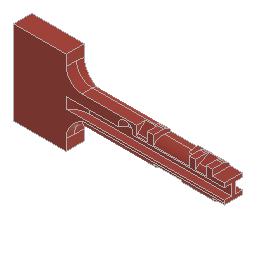
exec (Autodesk Fusion 360 design; units mm, degrees)
Autodesk Fusion 360 part; units mm, degrees
sketch "profile" plane through (0, 0, 0) normal (1, 0, 0) x (0, 1, 0)
  line L0 (0, 0) -> (1.725, 0) construction
  line L1 (1.725, 0) -> (1.725, 2.975) construction
  line L2 (0, 0) -> (1.5, 1.5) construction
  line L3 (0, 0) -> (1.725, 0) construction
  line L4 (1.725, 2.975) -> (1.725, 5.95) construction
  line L5 (1.725, 5.95) -> (3.45, 5.95) construction
  line L6 (3.45, 5.95) -> (1.95, 4.45) construction
  line L7 (1.725, 2.975) -> (1.375, 2.975) construction
  line L8 (1.375, 2.975) -> (1.375, 4)
  line L9 (1.725, 2.975) -> (2.075, 2.975) construction
  line L10 (1.375, 2.975) -> (1.375, 1.95)
  line L11 (2.075, 2.975) -> (2.075, 4)
  line L12 (2.075, 2.975) -> (2.075, 1.95)
  line L13 (1.375, 4) -> (0, 4)
  line L14 (1.375, 1.95) -> (0, 1.95)
  line L15 (2.075, 4) -> (3.45, 4)
  line L16 (2.075, 1.95) -> (3.45, 1.95)
  line L17 (3.45, 1.95) -> (3.45, 0)
  line L18 (0, 4) -> (0, 5.95)
  arc A0 (0, 1.5) -> (1.5, 0) centre (1.5, 1.5) ccw
  line L19 (0, 1.95) -> (0, 1.5)
  line L20 (1.5, 0) -> (3.45, 0)
  arc A1 (3.45, 4.45) -> (1.95, 5.95) centre (1.95, 4.45) ccw
  line L21 (1.95, 5.95) -> (0, 5.95)
  line L22 (3.45, 4.45) -> (3.45, 4)
  dimension "d1" = 1.725
  dimension "d2" = 2.975
  dimension "d3" = 45
  dimension "d4" = 2.1213
  dimension "d5" = 2.975
  dimension "d6" = 1.725
  dimension "d7" = 0.35
  dimension "d8" = 1.025
  dimension "d9" = 1.375
  constraint coincident L0.start L2.start
  constraint horizontal L0
  constraint perpendicular L0 L1
  constraint horizontal L3
  constraint parallel L1 L4
  constraint perpendicular L4 L5
  constraint equal L2 L6
  constraint parallel L2 L6
  constraint perpendicular L1 L7
  constraint perpendicular L7 L8
  constraint perpendicular L4 L9
  constraint equal L7 L9
  constraint perpendicular L7 L10
  constraint perpendicular L9 L11
  constraint perpendicular L9 L12
  constraint equal L8 L10
  constraint equal L10 L12
  constraint equal L11 L12
  constraint perpendicular L8 L13
  constraint perpendicular L10 L14
  constraint perpendicular L11 L15
  constraint perpendicular L12 L16
  constraint perpendicular L3 L17
  constraint perpendicular L5 L18
  constraint coincident L3 A0.end
  constraint coincident L2.end A0.centre
  constraint tangent A0 L19
  constraint tangent A0 L20
  constraint coincident L5 A1.end
  constraint coincident L6.end A1.centre
  constraint tangent A1 L21
  constraint tangent A1 L22
  constraint equal L13 L15
  constraint equal L15 L16
  constraint equal L14 L16
  constraint perpendicular L15 L22
  constraint parallel L20 L21
  measures "d1" distance of L0.start L0.end
  measures "d2" distance of L0.end L1.end
  measures "d3" angle of L2 L3
  measures "d4" distance of L0.start L2.end
  measures "d5" distance of L1.end L4.end
  measures "d6" distance of L4.end L5.end
  measures "d7" distance of L1.end L7.end
  measures "d8" distance of L7.end L8.end
  measures "d9" distance of L8.end L13.end
extrude "Extrude1" add sketch "profile" against normal blind 30
ref_plane "WorkPlane2" through (-30, 0, 0) normal (1, 0, 0) x (0, 1, 0)
sketch "bow" plane through (-30, 0, 0) normal (1, 0, 0) x (0, 1, 0)
  line L0 (0, 0) -> (0, -5.025)
  line L1 (0, 0) -> (0, 10.975)
  line L2 (0, 10.975) -> (3.45, 10.975)
  line L3 (3.45, 10.975) -> (3.45, -5.025)
  line L4 (3.45, -5.025) -> (0, -5.025)
  dimension "d91" = 5.025
  dimension "d92" = 10.975
  dimension "d93" = 3.45
  constraint coincident L0.start L1.start
  constraint vertical L0
  constraint parallel L0 L1
  constraint perpendicular L1 L2
  constraint perpendicular L2 L3
  constraint perpendicular L0 L4
  measures "d91" distance of L0.start L0.end
  measures "d92" distance of L0.start L1.end
  measures "d93" distance of L1.end L2.end
ref_plane "WorkPlane1" through (-15, 1.725, 4.975) normal (0, -1, 0) x (0, 0, 1)
sketch "dss dimples" plane through (0, 1.725, 0) normal (0, -1, 0) x (-1, 0, 0)
  line L0 (0, 0) -> (0, -2.975) construction
  line L1 (0, -2.975) -> (18.775, -2.975) construction
  line L2 (18.775, -2.975) -> (18.775, -4.275) construction
  line L3 (18.775, -2.975) -> (18.775, -1.675) construction
  circle A0 centre (18.775, -4.275) radius 0.4
  circle A1 centre (18.775, -1.675) radius 0.4
  dimension "d12" = 2.975
  dimension "d13" = 18.775
  dimension "d14" = 1.3
  dimension "d15" = 0.8
  constraint coincident L0.start origin
  constraint vertical L0
  constraint perpendicular L0 L1
  constraint perpendicular L1 L2
  constraint perpendicular L1 L3
  constraint equal L2 L3
  constraint coincident L2.end A0.centre
  constraint coincident L3.end A1.centre
  constraint equal A0 A1
  measures "d12" distance of L0.start L0.end
  measures "d13" distance of L0.end L1.end
  measures "d14" distance of L1.end L2.end
  measures "d15" diameter of A0
sketch "tip warding" plane through (0, 0, 0) normal (1, 0, 0) x (0, 1, 0)
  line L0 (0, 0) -> (3.45, 0)
  line L1 (3.45, 0) -> (3.45, 1.15)
  line L2 (3.45, 1.15) -> (0, 1.15)
  line L3 (0, 1.15) -> (0, 0)
  line L4 (0, 1.15) -> (0, 4.8) construction
  line L5 (0, 4.8) -> (0, 5.95)
  line L6 (0, 5.95) -> (3.45, 5.95)
  line L7 (3.45, 5.95) -> (3.45, 4.8)
  line L8 (3.45, 4.8) -> (0, 4.8)
  dimension "d16" = 3.45
  dimension "d17" = 1.15
  dimension "d18" = 3.65
  dimension "d19" = 1.15
  dimension "d20" = 3.45
  constraint coincident L0.start L3.end
  constraint horizontal L0
  constraint perpendicular L0 L1
  constraint perpendicular L1 L2
  constraint perpendicular L0 L3
  constraint perpendicular L2 L4
  constraint parallel L4 L5
  constraint perpendicular L5 L6
  constraint perpendicular L6 L7
  constraint perpendicular L5 L8
  measures "d16" distance of L0.start L0.end
  measures "d17" distance of L0.end L1.end
  measures "d18" distance of L2.end L4.end
  measures "d19" distance of L4.end L5.end
  measures "d20" distance of L5.end L6.end
sketch "1 cut" plane through (0, 0, 0) normal (1, 0, 0) x (0, 1, 0)
  line L0 (0, 0) -> (1.725, 0) construction
  line L1 (1.725, 0) -> (1.725, 2.975) construction
  line L2 (1.725, 2.975) -> (3.15, 5.4432) construction
  line L3 (1.725, 2.975) -> (5.325, 2.975) construction
  line L4 (1.725, 2.975) -> (0.3, 0.5068) construction
  line L5 (3.15, 5.4432) -> (5.0548, 4.3435)
  line L6 (3.15, 5.4432) -> (1.2452, 6.5429)
  line L7 (0.3, 0.5068) -> (2.2048, -0.5929)
  line L8 (0.3, 0.5068) -> (-1.6048, 1.6065)
  arc A0 (2.2048, -0.5929) -> (5.0548, 4.3435) centre (1.725, 2.975) ccw
  arc A1 (1.2452, 6.5429) -> (-1.6048, 1.6065) centre (1.725, 2.975) ccw
  circle A2 centre (1.725, 2.975) radius 4.25
  dimension "d21" = 1.725
  dimension "d22" = 2.975
  dimension "d23" = 2.85
  dimension "d24" = 60
  dimension "d25" = 3.6
  dimension "d26" = 8.5
  constraint coincident L0.start origin
  constraint horizontal L0
  constraint perpendicular L0 L1
  constraint horizontal L3
  constraint parallel L2 L4
  constraint equal L2 L4
  constraint perpendicular L2 L5
  constraint perpendicular L2 L6
  constraint perpendicular L4 L7
  constraint perpendicular L4 L8
  constraint coincident L1.end L2.start
  constraint coincident L7.end A0.start
  constraint coincident L3.end A0
  constraint equal L5 L6
  constraint equal L6 L8
  constraint equal A0 A1
  constraint concentric A1 A2
  measures "d21" distance of L0.start L0.end
  measures "d22" distance of L0.end L1.end
  measures "d23" distance of L1.end L2.end
  measures "d24" angle of L2 L3
  measures "d25" radius of A0
  measures "d26" diameter of A2
sketch "2 cut" plane through (0, 0, 0) normal (1, 0, 0) x (0, 1, 0)
  line L0 (0, 0) -> (1.725, 0) construction
  line L1 (1.725, 0) -> (1.725, 2.975) construction
  line L2 (1.725, 2.975) -> (-0.1513, 3.9726) construction
  line L3 (1.725, 2.975) -> (-0.1513, 2.975) construction
  line L4 (1.725, 2.975) -> (3.6013, 1.9774) construction
  line L5 (-0.1513, 3.9726) -> (1.213, 6.5384)
  line L6 (3.6013, 1.9774) -> (2.237, -0.5884)
  arc A0 (3.6013, 6.0474) -> (1.213, 6.5384) centre (1.725, 2.975) ccw
  line L7 (3.6013, 1.9774) -> (3.6013, 6.0474)
  arc A1 (-0.1513, -0.0974) -> (2.237, -0.5884) centre (1.725, 2.975) ccw
  line L8 (-0.1513, 3.9726) -> (-0.1513, -0.0974)
  circle A2 centre (1.725, 2.975) radius 4.25
  dimension "d27" = 1.725
  dimension "d28" = 2.975
  dimension "d29" = 28
  dimension "d30" = 2.125
  dimension "d31" = 3.6
  dimension "d32" = 8.5
  constraint coincident L0.start origin
  constraint horizontal L0
  constraint perpendicular L0 L1
  constraint horizontal L3
  constraint parallel L2 L4
  constraint equal L2 L4
  constraint perpendicular L2 L5
  constraint perpendicular L4 L6
  constraint equal L5 L6
  constraint coincident L1.end L2.start
  constraint vertical L7
  constraint coincident A0.start L7.end
  constraint perpendicular L3 L8
  constraint coincident A1.start L8.end
  constraint coincident L3.end L8
  constraint concentric A1 A2
  measures "d27" distance of L0.start L0.end
  measures "d28" distance of L0.end L1.end
  measures "d29" angle of L2 L3
  measures "d30" distance of L1.end L2.end
  measures "d31" radius of A0
  measures "d32" diameter of A2
sketch "3 cut" plane through (0, 0, 0) normal (1, 0, 0) x (0, 1, 0)
  line L0 (0, 0) -> (1.725, 0) construction
  line L1 (1.725, 0) -> (1.725, 2.975) construction
  line L2 (1.725, 2.975) -> (0.2489, 4.5036) construction
  line L3 (1.725, 2.975) -> (-0.4, 2.975) construction
  line L4 (0.2489, 4.5036) -> (2.3392, 6.5222)
  line L5 (1.725, 2.975) -> (3.2011, 1.4464) construction
  line L6 (3.2011, 1.4464) -> (1.1108, -0.5722)
  arc A0 (0.2489, 4.5036) -> (-0.4, 2.975) centre (1.725, 2.975) ccw
  arc A1 (3.2011, 1.4464) -> (3.85, 2.975) centre (1.725, 2.975) ccw
  arc A2 (3.85, 5.8809) -> (2.3392, 6.5222) centre (1.725, 2.975) ccw
  line L7 (3.85, 2.975) -> (3.85, 5.8809)
  arc A3 (-0.4, 0.0691) -> (1.1108, -0.5722) centre (1.725, 2.975) ccw
  line L8 (-0.4, 2.975) -> (-0.4, 0.0691)
  circle A4 centre (1.725, 2.975) radius 4.25
  dimension "d33" = 1.725
  dimension "d34" = 2.975
  dimension "d35" = 46
  dimension "d36" = 2.125
  dimension "d37" = 3.6
  dimension "d38" = 8.5
  constraint coincident L0.start origin
  constraint horizontal L0
  constraint perpendicular L0 L1
  constraint horizontal L3
  constraint perpendicular L2 L4
  constraint parallel L2 L5
  constraint equal L2 L5
  constraint perpendicular L5 L6
  constraint equal L4 L6
  constraint coincident L1.end L2.start
  constraint collinear L1.end L3.end A1.end
  constraint tangent A1 L7
  constraint coincident A2.start L7.end
  constraint tangent A0 L8
  constraint coincident A3.start L8.end
  constraint concentric A0 A4
  measures "d33" distance of L0.start L0.end
  measures "d34" distance of L0.end L1.end
  measures "d35" angle of L2 L3
  measures "d36" distance of L1.end L2.end
  measures "d37" radius of A2
  measures "d38" diameter of A4
sketch "4 cut" plane through (0, 0, 0) normal (1, 0, 0) x (0, 1, 0)
  line L0 (0, 0) -> (1.725, 0) construction
  line L1 (1.725, 0) -> (1.725, 2.975) construction
  line L2 (1.725, 2.975) -> (0.7935, 4.8849) construction
  line L3 (1.725, 2.975) -> (-0.4, 2.975) construction
  line L4 (1.725, 2.975) -> (2.6565, 1.0651) construction
  line L5 (0.7935, 4.8849) -> (3.4053, 6.1588)
  line L6 (2.6565, 1.0651) -> (0.0447, -0.2088)
  arc A0 (0.7935, 4.8849) -> (-0.4, 2.975) centre (1.725, 2.975) ccw
  arc A1 (2.6565, 1.0651) -> (3.85, 2.975) centre (1.725, 2.975) ccw
  arc A2 (3.85, 5.8809) -> (3.4053, 6.1588) centre (1.725, 2.975) ccw
  line L7 (3.85, 2.975) -> (3.85, 5.8809)
  arc A3 (-0.4, 0.0691) -> (0.0447, -0.2088) centre (1.725, 2.975) ccw
  line L8 (-0.4, 2.975) -> (-0.4, 0.0691)
  circle A4 centre (1.725, 2.975) radius 4.25
  dimension "d39" = 1.725
  dimension "d40" = 2.975
  dimension "d41" = 64
  dimension "d42" = 2.125
  dimension "d43" = 3.6
  dimension "d44" = 8.5
  constraint coincident L0.start origin
  constraint horizontal L0
  constraint perpendicular L0 L1
  constraint horizontal L3
  constraint parallel L2 L4
  constraint equal L2 L4
  constraint perpendicular L2 L5
  constraint perpendicular L4 L6
  constraint equal L5 L6
  constraint coincident L1.end L2.start
  constraint collinear L1.end L3.end A1.end
  constraint tangent A1 L7
  constraint coincident A2.start L7.end
  constraint tangent A0 L8
  constraint coincident A3.start L8.end
  constraint concentric A1 A4
  measures "d39" distance of L0.start L0.end
  measures "d40" distance of L0.end L1.end
  measures "d41" angle of L2 L3
  measures "d42" distance of L1.end L2.end
  measures "d43" radius of A2
  measures "d44" diameter of A4
sketch "5 cut" plane through (0, 0, 0) normal (1, 0, 0) x (0, 1, 0)
  line L0 (0, 0) -> (1.725, 0) construction
  line L1 (1.725, 0) -> (1.725, 2.975) construction
  line L2 (1.725, 2.975) -> (1.4293, 5.0793) construction
  line L3 (1.725, 2.975) -> (-0.4, 2.975) construction
  line L4 (1.725, 2.975) -> (2.0207, 0.8707) construction
  line L5 (1.4293, 5.0793) -> (3.85, 5.4195)
  line L6 (2.0207, 0.8707) -> (-0.4, 0.5305)
  arc A0 (1.4293, 5.0793) -> (-0.4, 2.975) centre (1.725, 2.975) ccw
  arc A1 (2.0207, 0.8707) -> (3.85, 2.975) centre (1.725, 2.975) ccw
  line L7 (3.85, 2.975) -> (3.85, 5.4195)
  line L8 (-0.4, 0.5305) -> (-0.4, 2.975)
  circle A2 centre (1.725, 2.975) radius 4.25
  dimension "d45" = 1.725
  dimension "d46" = 2.975
  dimension "d47" = 82
  dimension "d48" = 2.125
  dimension "d49" = 8.5
  constraint coincident L0.start origin
  constraint horizontal L0
  constraint perpendicular L0 L1
  constraint horizontal L3
  constraint parallel L2 L4
  constraint equal L2 L4
  constraint perpendicular L2 L5
  constraint perpendicular L4 L6
  constraint equal L5 L6
  constraint coincident L1.end L2.start
  constraint collinear L1.end L3.end A1.end
  constraint coincident L5.end L7.end
  constraint tangent A0 L8
  constraint concentric A1 A2
  measures "d45" distance of L0.start L0.end
  measures "d46" distance of L0.end L1.end
  measures "d47" angle of L2 L3
  measures "d48" distance of L1.end L2.end
  measures "d49" diameter of A2
sketch "6 cut" plane through (0, 0, 0) normal (1, 0, 0) x (0, 1, 0)
  line L0 (0, 0) -> (1.725, 0) construction
  line L1 (1.725, 0) -> (1.725, 2.975) construction
  line L2 (1.725, 2.975) -> (2.094, 5.0677) construction
  line L3 (1.725, 2.975) -> (-0.4, 2.975) construction
  line L4 (1.725, 2.975) -> (1.356, 0.8823) construction
  line L5 (2.094, 5.0677) -> (3.85, 4.7581)
  line L6 (1.356, 0.8823) -> (-0.4, 1.1919)
  arc A0 (2.094, 5.0677) -> (-0.4, 2.975) centre (1.725, 2.975) ccw
  arc A1 (1.356, 0.8823) -> (3.85, 2.975) centre (1.725, 2.975) ccw
  line L7 (3.85, 2.975) -> (3.85, 4.7581)
  line L8 (-0.4, 1.1919) -> (-0.4, 2.975)
  circle A2 centre (1.725, 2.975) radius 4.25
  dimension "d50" = 1.725
  dimension "d51" = 2.975
  dimension "d52" = 100
  dimension "d53" = 2.125
  dimension "d54" = 8.5
  constraint coincident L0.start origin
  constraint horizontal L0
  constraint perpendicular L0 L1
  constraint horizontal L3
  constraint parallel L2 L4
  constraint equal L2 L4
  constraint perpendicular L2 L5
  constraint perpendicular L4 L6
  constraint equal L5 L6
  constraint coincident L1.end L2.start
  constraint collinear L1.end L3.end A1.end
  constraint coincident L5.end L7.end
  constraint tangent A0 L8
  constraint concentric A1 A2
  measures "d50" distance of L0.start L0.end
  measures "d51" distance of L0.end L1.end
  measures "d52" angle of L2 L3
  measures "d53" distance of L1.end L2.end
  measures "d54" diameter of A2
extrude "Extrude14" add sketch "bow" against normal blind 10
fillet "Fillet1" radius 3 4 edges at (-30, 0.975, 5.95) (-30, 3.0107, 5.5107) (-30, 2.475, 0) (-30, 0.4393, 0.4393)
fillet "Fillet2" radius 4 2 edges at (-30, 1.375, 2.975) (-30, 2.075, 2.975)
extrude "Extrude2" cut sketch "dss dimples" against normal blind 1 draft 45 from surface at -0.725 contours A1
extrude "Extrude3" cut sketch "dss dimples" along normal blind 1 draft 45 from surface at 0.725 contours A0
extrude "tip cut" cut sketch "tip warding" against normal blind 2.25
extrude "1" cut sketch "1 cut" along normal mid plane 2.05 from surface at -2.825
extrude "2" cut sketch "4 cut" along normal mid plane 2.05 from surface at -4.425
extrude "3" cut sketch "1 cut" along normal mid plane 2.05 from surface at -6.025
extrude "4" cut sketch "5 cut" along normal mid plane 2.05 from surface at -7.625
extrude "5" cut sketch "6 cut" along normal mid plane 2.05 from surface at -9.225
extrude "6" cut sketch "6 cut" along normal mid plane 2.05 from surface at -10.825
extrude "7" cut sketch "6 cut" along normal mid plane 2.05 from surface at -12.425
extrude "8" cut sketch "1 cut" along normal mid plane 2.05 from surface at -14.025
extrude "9" cut sketch "3 cut" along normal mid plane 2.05 from surface at -15.625
equation "d1 = 3.45 mm * 0.5"
equation "d2 = 5.95 mm * 0.5"
equation "d4 = ( sqrt(1.5 ^ 2 + 1.5 ^ 2) ) * 1 mm"
equation "d5 = d2"
equation "d6 = d1"
equation "d7 = ( 0.7 / 2 ) * 1 mm"
equation "d8 = ( 2.05 / 2 ) * 1 mm"
equation "d9 = d1 - d7"
equation "d10 = -30 mm"
equation "d12 = d2"
equation "d13 = 17 mm + 1 mm + ( ( 1.55 / 2 ) * 1 mm )"
equation "d16 = d1 * 2"
equation "d17 = d2 - 1.825 mm"
equation "d18 = ( d2 - d17 ) * 2"
equation "d19 = d17"
equation "d20 = d1 * 2"
equation "d21 = d1"
equation "d22 = d2"
equation "d27 = d1"
equation "d28 = d2"
equation "d30 = ( 4.25 / 2 ) * 1 mm"
equation "d33 = d1"
equation "d34 = d2"
equation "d36 = ( 4.25 / 2 ) * 1 mm"
equation "d39 = d1"
equation "d40 = d2"
equation "d42 = ( 4.25 / 2 ) * 1 mm"
equation "d45 = d1"
equation "d46 = d2"
equation "d48 = ( 4.25 / 2 ) * 1 mm"
equation "d50 = d1"
equation "d51 = d2"
equation "d53 = ( 4.25 / 2 ) * 1 mm"
equation "d55 = -0.725 mm"
equation "d56 = -1 mm"
equation "d57 = 45 deg"
equation "d58 = -d55"
equation "d59 = -d56"
equation "d60 = d57"
equation "d63 = -1.225 mm - ( 1.6 * 1 mm )"
equation "d66 = -1.225 mm - ( 1.6 * 2 mm )"
equation "d69 = -1.225 mm - ( 1.6 * 3 mm )"
equation "d72 = -1.225 mm - ( 1.6 * 4 mm )"
equation "d75 = -1.225 mm - ( 1.6 * 5 mm )"
equation "d78 = -1.225 mm - ( 1.6 * 6 mm )"
equation "d81 = -1.225 mm - ( 1.6 * 7 mm )"
equation "d84 = -1.225 mm - ( 1.6 * 8 mm )"
equation "d87 = -1.225 mm - ( 1.6 * 9 mm )"
equation "d90 = d10"
equation "d91 = 8 mm - d2"
equation "d92 = d2 * 2 + d91"
equation "d93 = d1 * 2"
